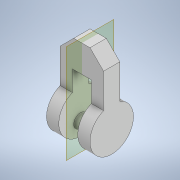
# Autodesk Inventor part: 2번부품
Saved by Autodesk Inventor 2022 (Build 260153000, 153)
## iProperties
Created: 2021-09-04
Part Number: 2번부품
Material: 일반
Document SubType Name: Modeling
Designer: 서울공업고등학교
Density: 1 g/cm^3
Appearance: 기본값
Author: 서울공업고등학교
Autodesk Inventor part; units mm, degrees
ref_plane "YZ Plane" through (0, 0, 0) normal (1, 0, 0) x (0, 1, 0)
ref_plane "XZ Plane" through (0, 0, 0) normal (0, 1, 0) x (-1, 0, 0)
sketch "스케치1" plane through (0, 0, 0) normal (0, 0, 1) x (1, 0, 0)
  line L0 (0, 0) -> (0, -28)
  line L1 (0, -28) -> (4.5, -28)
  line L2 (4.5, -26.5) -> (4.5, -10)
  line L3 (4.5, -10) -> (8, -10)
  line L4 (8, -10) -> (8, 0)
  line L5 (8, 0) -> (0, 0)
  line L6 (4.5, -28) -> (4.5, -26.5)
  dimension "d0" = 28
  dimension "d1" = 10
  dimension "d6" = 8
  constraints: 14 end point, 3 perpendicular, 2 vertical
  measures "d0" distance of L0.start L0.end
  measures "d1" distance between parallel lines of L3 L5
  measures "d6" distance between parallel lines of L4 L0
extrude "돌출1" add sketch "스케치1" along normal mid plane 6
mirror "미러1" about plane through (8, -10, 0) normal (1, 0, 0) of "돌출1"
chamfer "모따기1" distance 5 angle 45 1 edges at (0, 0, 0)
chamfer "모따기2" distance 5 angle 45 1 edges at (16, 0, 0)
sketch "스케치2" plane through (0, -28, -3) normal (-1, 0, 0) x (0, 0, 1)
  circle A0 centre (3, 3) radius 8
  line L0 (0, 0) -> (6, 0) projected
  point P0 (3, 28)
  dimension "d15" = 16
  dimension "d16" = 3
  constraints: 1 centre point
  measures "d15" diameter of A0
  measures "d16" distance from line of L0 A0.centre
extrude "돌출2" add sketch "스케치2" against normal blind 4.5
ref_plane "작업 평면1" through (8, -10, 3) normal (1, 0, 0) x (0, 0, -1)
mirror "미러2" about plane through (8, -10, 3) normal (1, 0, 0) of "돌출2"
sketch "스케치3" plane through (4.5, -10, 3) normal (1, 0, 0) x (0, 0, -1)
  circle A0 centre (3, -18) radius 2.5
  line L0 (6, 10) -> (6, 5) projected
  point P0 (3, 10)
  dimension "d19" = 5
  dimension "d20" = 28
  dimension "d21" = 3
  constraints: 1 centre point
  measures "d19" diameter of A0
  measures "d20" distance of point (3, 10) A0.centre
  measures "d21" distance from line of L0 A0.centre
extrude "돌출3" add sketch "스케치3" along normal blind 7
ref_plane "작업 평면2" through (8, -10, 3) normal (1, 0, 0) x (0, 0, -1)
